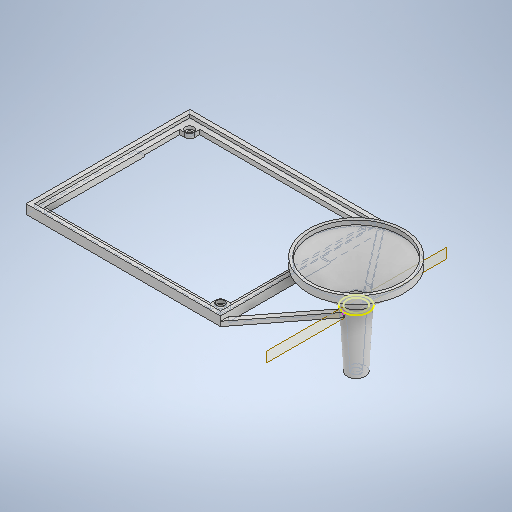
# Autodesk Inventor part: ResoarHållare
Saved by Autodesk Inventor 2025.2 (Build 292293000, 293)
## iProperties
Created: 2025-01-28
Part Number: ResoarHållare
Material: Generic
Document SubType Name: Modeling
Designer: 24oscnor
Density: 1 g/cm^3
Appearance: Default
Author: 24oscnor
Autodesk Inventor part; units mm, degrees
ref_plane "YZ Plane" through (0, 0, 0) normal (1, 0, 0) x (0, 1, 0)
ref_plane "XZ Plane" through (0, 0, 0) normal (0, 1, 0) x (-1, 0, 0)
ref_plane "XY Plane" through (0, 0, 0) normal (0, 0, 1) x (1, 0, 0)
sketch "Sketch1" plane through (0, 0, 0) normal (0, 1, 0) x (-1, 0, 0)
  line L0 (0, 0) -> (120, 0)
  line L1 (120, 0) -> (120, -100)
  line L2 (120, -100) -> (0, -100)
  line L3 (0, -100) -> (0, 0)
  line L4 (117, -97) -> (117, -3)
  line L5 (117, -3) -> (3, -3)
  line L6 (3, -3) -> (3, -97)
  line L7 (3, -97) -> (117, -97)
  line L8 (123, -103) -> (123, 3)
  line L9 (123, 3) -> (-3, 3)
  line L10 (-3, 3) -> (-3, -103)
  line L11 (-3, -103) -> (123, -103)
  line L12 (120.25, -100.25) -> (120.25, 0.25)
  line L13 (120.25, 0.25) -> (-0.25, 0.25)
  line L14 (-0.25, 0.25) -> (-0.25, -100.25)
  line L15 (-0.25, -100.25) -> (120.25, -100.25)
  circle A0 centre (6.25, -6.25) radius 3.25
  line L16 (9.5, -6.25) -> (9.5, -3)
  line L17 (6.25, -9.5) -> (3, -9.5)
  circle A1 centre (113.75, -93.75) radius 3.25
  line L18 (113.75, -90.5) -> (117, -90.5)
  line L19 (110.5, -93.75) -> (110.5, -97)
  dimension "d0" = 120
  dimension "d1" = 100
  dimension "d2" = 3
  dimension "d3" = 3
  dimension "d4" = 0.25
  dimension "d9" = 6.5
  dimension "d10" = 3.25
  dimension "d11" = 3.25
  dimension "d12" = 3.25
  dimension "d13" = 6.5
  dimension "d14" = 3.25
  dimension "d15" = 3.25
  constraints: 40 end point, 8 parallel, 8 perpendicular, 4 point on circle, 4 point on line, 3 tangent, 2 centre point, 1 horizontal, 9 other
  measures "d0" distance of L1.end L2.end
  measures "d1" distance of L2.end L0.start
  measures "d2" distance between parallel lines of L1 L4
  measures "d3" distance between parallel lines of L8 L1
  measures "d4" distance between parallel lines of L12 L1
  measures "d9" diameter of A0
  measures "d10" distance from line of L5 A0.centre
  measures "d11" distance of L17.start L17.end
  measures "d12" distance of L16.start L16.end
  measures "d13" diameter of A1
  measures "d14" distance from line of L7 A1.centre
  measures "d15" distance of L18.start L18.end
extrude "Extrusion1" add sketch "Sketch1" along normal blind 3 contours L0 L1 L2 L3 | L7 A1 L4 | A1 L18 L4 | A1 | L7 L19 A1 | L16 A0 L5 | L6 A0 L17 | A0 L6 L5 | A0 | L15 L14 L13 L12
extrude "Extrusion2" add sketch "Sketch1" along normal blind 5 contours L11 L10 L9 L8
sketch "Sketch2" plane through (0, 0, 0) normal (0, -1, 0) x (1, 0, 0)
  line L0 (3, -103) -> (-123, -103) construction
  line L1 (-60, -103) -> (-60, 3.5996) construction
  line L2 (-3, -97) -> (-3, -9.5) projected
  line L3 (3, -103) -> (-3, -103)
  line L4 (-3, -103) -> (-3, -68)
  line L5 (-3, -68) -> (3, -68)
  line L6 (3, -68) -> (3, -103)
  line L7 (-3, -97) -> (-60, -97)
  line L8 (-60, -97) -> (-60, -103)
  line L9 (-60, -103) -> (-3, -103)
  line L10 (-3, -103) -> (-3, -97)
  line L11 (-123, -103) -> (3, -103) construction
  line L12 (-117, -97) -> (-117, -9.5)
  line L13 (-123, -103) -> (-117, -103)
  line L14 (-117, -103) -> (-117, -68)
  line L15 (-117, -68) -> (-123, -68)
  line L16 (-123, -68) -> (-123, -103)
  line L17 (-117, -97) -> (-60, -97)
  line L18 (-60, -103) -> (-117, -103)
  line L19 (-117, -103) -> (-117, -97)
  circle A0 centre (-113.75, -93.75) radius 3.25
  line L20 (-117, -90.5) -> (-113.75, -90.5) projected
  line L21 (-117, -90.5) -> (-113.75, -90.5)
  line L22 (-110.5, -93.75) -> (-110.5, -97)
  line L23 (-123, -68) -> (-117, -68)
  line L24 (-117, -68) -> (-117, 3)
  line L25 (-117, 3) -> (-123, 3)
  line L26 (-123, 3) -> (-123, -68)
  line L27 (-9.5, -3) -> (-117, -3) projected
  line L28 (-123, 3) -> (3, 3) projected
  line L29 (-117, -3) -> (3, -3)
  line L30 (3, -3) -> (3, 3)
  line L31 (3, 3) -> (-117, 3)
  line L32 (-117, 3) -> (-117, -3)
  line L33 (-3, -68) -> (3, -68)
  line L34 (3, -68) -> (3, -3)
  line L35 (3, -3) -> (-3, -3)
  line L36 (-3, -3) -> (-3, -68)
  circle A1 centre (-6.25, -6.25) radius 3.25
  arc A2 (-9.5, -6.25) -> (-6.25, -9.5) centre (-6.25, -6.25) ccw projected
  line L37 (-3, -9.5) -> (-6.25, -9.5)
  line L38 (-9.5, -6.25) -> (-9.5, -3)
  point P0 (0, 0)
  point P1 (-117, 3)
  point P2 (-117, -9.5)
  dimension "d16" = 35
  dimension "d17" = 6.5
  dimension "d18" = 3.25
  dimension "d19" = 3.25
  dimension "d20" = 3.25
  dimension "d21" = 106.5996
  dimension "d67" = 0
  dimension "d68" = 0
  dimension "d69" = 0
  dimension "d70" = 6.5
  constraints: 68 end point, 11 equal length, 8 perpendicular, 8 symmetric about line, 5 horizontal, 3 point on line, 2 centre point, 2 point on circle, 1 midpoint, 1 tangent, 1 vertical
  measures "d16" distance of L5.end L0.start
  measures "d17" diameter of A0
  measures "d18" distance from line of L12 A0.centre
  measures "d19" distance from line of L17 A0.centre
  measures "d20" distance of L22.start L22.end
  measures "d21" distance of L1.start L1.end
  measures "d67" distance between parallel lines of L28 L25
  measures "d68" distance of A2.centre A1.centre
  measures "d69" distance of A2.centre A1.centre
  measures "d70" diameter of A1
extrude "Extrusion3" add sketch "Sketch2" along normal blind 1 contours L2 L36 L29 L34 L5 | L37 A1 L36 | A1 L29 L36 | A1 | L29 L27 L24 L28 L30 | A1 L38 L29 | L24 L12 L15 L26 L25
ref_plane "Work Plane1" through (38, 0, 3) normal (1, 0, 0) x (0, 0, -1)
sketch "Sketch3" plane through (38, 0, 3) normal (1, 0, 0) x (0, 0, -1)
  line L0 (53, -10.8881) -> (53, 16.7673)
  line L1 (106, 5) -> (0, 5) construction
  line L2 (106, 0) -> (106, 5) construction
  line L3 (106, 5) -> (106, -1) construction
  line L4 (45, 5) -> (22.0187, 24.2836)
  line L5 (45, 5) -> (47.0963, -35)
  line L6 (53, 5) -> (37.5678, 5) construction
  line L7 (50.0867, -34.7385) -> (47.9276, 6.4597)
  line L8 (47.9276, 6.4597) -> (23.947, 26.5818)
  line L9 (22.0187, 24.2836) -> (23.947, 26.5818)
  line L10 (22.0187, 24.2836) -> (22.0187, 29.2836)
  line L11 (22.0187, 29.2836) -> (23.947, 29.2836)
  line L12 (23.947, 29.2836) -> (23.947, 26.5818)
  line L13 (47.0963, -35) -> (50.1079, -35)
  line L14 (50.1079, -35) -> (50.0867, -34.7385)
  point P0 (3, 0)
  dimension "d26" = 106
  dimension "d27" = 16
  dimension "d28" = 30
  dimension "d29" = 93
  dimension "d30" = 40
  dimension "d31" = 40
  dimension "d32" = 3
  dimension "d34" = 3
  dimension "d37" = 5
  dimension "d48" = 0.2615
  dimension "d49" = 3.0116
  constraints: 26 end point, 3 vertical, 2 perpendicular, 2 point on line, 1 horizontal, 1 midpoint, 1 other
  measures "d26" diameter of L2 L0
  measures "d27" diameter of L4.start L0
  measures "d28" distance of L4.start L4.end
  measures "d29" angle of L5 L1
  measures "d30" angle of L4 L1
  measures "d31" vertical distance of L4.start L5.end
  measures "d32" distance between parallel lines of L5 L7
  measures "d34" distance of L4.end L8.end
  measures "d37" distance of L4.end L10.end
  measures "d48" vertical distance of L13.end L7.start
  measures "d49" distance of L5.end L13.end
revolve "Revolution1" add sketch "Sketch3" angle 360 about axis through (38, -10.8881, -50) along (0, 1, 0)
sketch "Sketch4" plane through (0, 0, 0) normal (0, 1, 0) x (-1, 0, 0)
  line L0 (-3, -68) -> (-3, -103) projected
  circle A0 centre (-38, -50) radius 8 projected
  line L1 (-3, -1.8865) -> (-3, 3)
  line L2 (-3, -103) -> (-3, -98.1135)
  circle A1 centre (-38, -50) radius 5.0724 projected
  circle A2 centre (-38, -50) radius 5.9037 projected
  line L3 (-38, -50) -> (-3, -50) construction
  line L4 (-3, -103) -> (-3, -98.1135) construction
  line L5 (-38.3984, -57.7256) -> (-35.0429, -57.1307) construction
  line L6 (-3, 3) -> (-3, -1.8865)
  line L7 (-3, 3) -> (-3, -1.8865) construction
  line L8 (-38.3984, -42.2744) -> (-35.0429, -42.8693) construction
  line L9 (-3, -103) -> (-38, -58)
  line L10 (-38, -42) -> (-3, 3)
  line L11 (-0.6319, -101.1582) -> (-35.6319, -56.1582)
  line L12 (-35.6319, -43.8418) -> (-0.6319, 1.1582)
  point P0 (0, 0)
  point P1 (-34.7396, -42.6945)
  point P2 (-34.7396, -57.3055)
  dimension "d74" = 3
  dimension "d75" = 3
  constraints: 24 end point, 3 symmetric about line, 2 collinear, 2 parallel, 2 point on circle, 2 point on line, 1 horizontal
  measures "d74" distance between parallel lines of L12 L10
  measures "d75" distance between parallel lines of L11 L9
extrude "Extrusion4" add sketch "Sketch4" along normal blind 2 contours L0 L9 A0 L11 | L10 L1 L12 A0
sketch "Sketch6" plane through (38, -35, -50) normal (0, -1, 0) x (1, 0, 0)
  circle A0 centre (0, 0) radius 2.9133 projected
  circle A1 centre (0, 0) radius 3
  point P0 (-38, 50)
  dimension "d50" = 6
  constraints: 1 centre point, 1 coincident
  measures "d50" diameter of A1
extrude "Extrusion6" cut sketch "Sketch6" against normal through all
sketch "Sketch7" plane through (0, 3, 0) normal (0, 1, 0) x (1, 0, 0)
  circle A0 centre (-113.75, 93.75) radius 2.75
  arc A1 (-113.75, 90.5) -> (-110.5, 93.75) centre (-113.75, 93.75) ccw projected
  circle A2 centre (-6.25, 6.25) radius 2.75
  arc A3 (-6.25, 9.5) -> (-9.5, 6.25) centre (-6.25, 6.25) ccw projected
  point P0 (0, 0)
  dimension "d53" = 5.5
  dimension "d54" = 0
  dimension "d55" = 0
  dimension "d56" = 5.5
  dimension "d57" = 0
  dimension "d58" = 0
  constraints: 2 centre point
  measures "d53" diameter of A0
  measures "d54" distance of A1.centre A0.centre
  measures "d55" distance of A1.centre A0.centre
  measures "d56" diameter of A2
  measures "d57" distance of A3.centre A2.centre
  measures "d58" distance of A3.centre A2.centre
extrude "Extrusion7" cut sketch "Sketch7" against normal blind 2
sketch "Sketch8" plane through (-6.25, 1, -6.25) normal (0, 1, 0) x (1, 0, 0)
  circle A0 centre (0, 0) radius 1.625
  circle A1 centre (0, 0) radius 2.75 projected
  circle A2 centre (-107.5, 87.5) radius 1.625
  circle A3 centre (-107.5, 87.5) radius 2.75 projected
  point P0 (6.25, -6.25)
  dimension "d61" = 3.25
  dimension "d62" = 1.125
  dimension "d63" = 3.25
  dimension "d64" = 1.125
  constraints: 2 centre point
  measures "d61" diameter of A0
  measures "d62" radial gap between concentric circles of A1 A0
  measures "d63" diameter of A2
  measures "d64" radial gap between concentric circles of A3 A2
extrude "Extrusion8" cut sketch "Sketch8" against normal blind 2 contours A0 | A2
sketch "Sketch9" plane through (0, 0, 0) normal (0, -1, 0) x (1, 0, 0)
  line L0 (3, -68) -> (-3, -68) projected
  line L1 (0, -68) -> (30.2222, -68)
  line L2 (3, -1.8865) -> (3, 3)
  line L3 (34.7396, -42.6945) -> (3, -1.8865) projected
  line L4 (3, -1.8865) -> (34.7396, -42.6945)
  line L5 (3, 3) -> (-123, 3) projected
  line L6 (3, 3) -> (38, -42)
  circle A0 centre (38, -50) radius 8 projected
  line L7 (38, -58) -> (3, -103) projected
  line L8 (30.2222, -68) -> (38, -58)
  line L9 (3, -98.1135) -> (34.7396, -57.3055) projected
  line L10 (34.7396, -57.3055) -> (26.4216, -68)
  point P0 (0, 0)
  constraints: 12 end point, 2 collinear, 2 point on line, 1 horizontal, 1 midpoint, 1 perpendicular, 1 point on circle
extrude "Extrusion9" add sketch "Sketch9" along normal blind 1 contours L9 A0 L7 L1 | L3 L2 L6 A0
sketch "Sketch11" plane through (0, 2, 0) normal (0, 1, 0) x (1, 0, 0)
  arc A0 (34.7396, 42.6945) -> (38, 42) centre (38, 50) ccw projected
  circle A1 centre (38, 50) radius 5.9037 projected
  circle A2 centre (38, 50) radius 8 projected
  point P0 (0, 0)
  point P1 (38.1855, 42.0022)
sketch "Sketch12" plane through (0, -1, 0) normal (0, -1, 0) x (1, 0, 0)
  arc A0 (38, -42) -> (34.7396, -42.6945) centre (38, -50) ccw projected
  line L0 (38, -42) -> (34.7396, -42)
  line L1 (34.7396, -42) -> (34.7396, -44.0733)
  line L2 (34.7396, -44.0733) -> (38, -44.0733)
  line L3 (38, -44.0733) -> (38, -42)
  circle A1 centre (38, -50) radius 8 construction
  line L4 (46, -50) -> (30, -50) construction
  line L5 (38, -58) -> (34.7396, -58)
  line L6 (34.7396, -58) -> (34.7396, -55.9267)
  line L7 (34.7396, -55.9267) -> (38, -55.9267)
  line L8 (38, -55.9267) -> (38, -58)
  point P0 (0, 0)
  dimension "d76" = 0
  constraints: 18 end point, 4 symmetric about line, 2 horizontal, 2 parallel, 2 point on circle, 1 perpendicular
  measures "d76" distance from line of A0.end L1
extrude "Extrusion10" add sketch "Sketch12" against normal blind 3 contours L3 L2 L1 A0 | L5 L6 L7 L8
body "Solid1"
